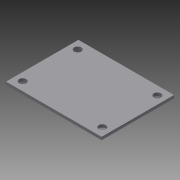
# Autodesk Inventor part: Swivel_Caster_Plate
Saved by Autodesk Inventor 2014 (Build 180170000, 170)
## iProperties
Created: 2016-08-26
Part Number: Swivel_Caster_Plate
Material: Generic
Document SubType Name: Modeling
Designer: jmw3
Density: 1 g/cm^3
Appearance: Default
Author: jmw3
Autodesk Inventor part; units mm, degrees
ref_plane "YZ Plane" through (0, 0, 0) normal (1, 0, 0) x (0, 1, 0)
ref_plane "XZ Plane" through (0, 0, 0) normal (0, 1, 0) x (-1, 0, 0)
ref_plane "XY Plane" through (0, 0, 0) normal (0, 0, 1) x (1, 0, 0)
sketch "Sketch1" plane through (0, 0, 0) normal (0, 1, 0) x (-1, 0, 0)
  line L0 (0, -55.5625) -> (0, 55.5625) projected
  line L1 (73.3425, 0) -> (-73.3425, 0) projected
  line L2 (52.3875, -39.6875) -> (-52.3875, -39.6875)
  line L3 (-52.3875, -39.6875) -> (-52.3875, 39.6875)
  line L4 (-52.3875, 39.6875) -> (52.3875, 39.6875)
  line L5 (52.3875, 39.6875) -> (52.3875, -39.6875)
  circle A0 centre (43.6562, -30.1625) radius 3.9688
  circle A1 centre (43.6562, 30.1625) radius 3.9688
  circle A2 centre (-43.6562, -30.1625) radius 3.9688
  circle A3 centre (-43.6562, 30.1625) radius 3.9688
  point P0 (0, 0)
  dimension "d0" = 104.775
  dimension "d1" = 79.375
  dimension "d4" = 7.9375
  dimension "d7" = 87.3125
  dimension "d8" = 60.325
  constraints: 8 end point, 4 centre point, 3 symmetric about line, 2 parallel, 1 horizontal, 1 perpendicular, 5 other
  measures "d0" distance of L3.end L4.end
  measures "d1" distance between parallel lines of L4 L2
  measures "d4" diameter of A0
  measures "d7" distance of A0.centre A2.centre
  measures "d8" distance of A0.centre A1.centre
extrude "Extrusion1" add sketch "Sketch1" along normal blind 3.175
body "Solid1"
